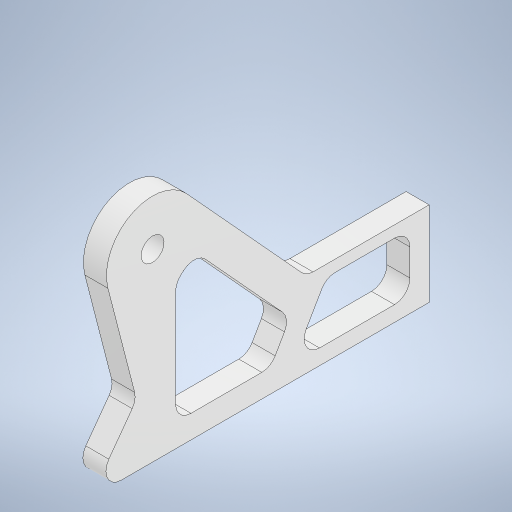
# Autodesk Inventor part: Upright
Saved by Autodesk Inventor 2023.2 (Build 272271000, 271)
## iProperties
Created: 2023-11-13
Part Number: Upright
Material: UHMW, White
Document SubType Name: Modeling
Designer: Nathan Cai
Density: 0.94 g/cm^3
Appearance: Smooth - White
Mass: 83.2223 g
Surface Area: 143.277 cm^2
Volume: 30.8231 cm^3
Author: Nathan Cai
Autodesk Inventor part; units mm, degrees
ref_plane "YZ Plane" through (0, 0, 0) normal (1, 0, 0) x (0, 1, 0)
ref_plane "XZ Plane" through (0, 0, 0) normal (0, 1, 0) x (-1, 0, 0)
ref_plane "XY Plane" through (0, 0, 0) normal (0, 0, 1) x (1, 0, 0)
sketch "Sketch1" plane through (0, 0, 0) normal (1, 0, 0) x (0, 1, 0)
  circle A0 centre (0, 0) radius 4.7625
  line L0 (0, 0) -> (-76.2, 0) construction
  circle A1 centre (0, 0) radius 19.05
  line L1 (-4.7625, 18.4451) -> (-76.2, 0)
  line L2 (-76.2, 0) -> (-76.2, -114.3)
  circle A2 centre (0, 0) radius 76.2 construction
  line L3 (-76.2, -114.3) -> (-41.275, -114.3)
  line L4 (-41.275, -114.3) -> (-41.275, -63.5)
  line L5 (-41.275, -63.5) -> (-76.2, -43.336)
  line L6 (-41.275, -63.5) -> (12.8474, -14.0658)
  line L7 (-52.8131, -56.8385) -> (-8.9789, -16.8012)
  line L8 (-66.675, -9.525) -> (-66.675, -48.8353)
  line L9 (-46.0375, -71.7489) -> (-76.2, -54.3346)
  line L10 (-46.0375, -71.7489) -> (-46.0375, -106.3625)
  line L11 (-46.0375, -106.3625) -> (-69.85, -106.3625)
  line L12 (-69.85, -106.3625) -> (-69.85, -58.0007)
  line L13 (-66.675, -9.525) -> (-64.7847, -9.525)
  line L14 (-64.7847, -9.525) -> (-16.4978, -9.525)
  line L15 (-76.2, 0) -> (-41.275, 0)
  line L16 (-41.275, 0) -> (-41.275, 25.4) construction
  line L17 (-41.275, 25.4) -> (-76.2, 25.4) construction
  line L18 (-76.2, 25.4) -> (-76.2, 0)
  line L19 (-41.275, 0) -> (-76.2, 25.4)
  point P0 (-50.4255, 6.6549)
  dimension "d0" = 9.525
  dimension "d1" = 76.2
  dimension "d2" = 38.1
  dimension "d3" = 114.3
  dimension "d4" = 152.4
  dimension "d5" = 34.925
  dimension "d6" = 50.8
  dimension "d7" = 60
  dimension "d9" = 12.7
  dimension "d10" = 9.525
  dimension "d11" = 9.525
  dimension "d12" = 7.9375
  dimension "d13" = 6.35
  dimension "d14" = 4.7625
  dimension "d17" = 9.525
  dimension "d19" = 34.925
  dimension "d20" = 25.4
  constraints: 40 end point, 6 parallel, 6 point on line, 4 point on circle, 3 centre point, 3 coincident, 3 horizontal, 3 perpendicular, 2 tangent, 1 vertical
  measures "d0" diameter of A0
  measures "d1" distance of L0.start L0.end
  measures "d2" diameter of A1
  measures "d3" distance of L0.end L2.end
  measures "d4" diameter of A2
  measures "d5" distance of L2.end L3.end
  measures "d6" distance of L3.end L4.end
  measures "d7" angle of L2 L5
  measures "d9" distance between parallel lines of L6 L7
  measures "d10" distance between parallel lines of L2 L8
  measures "d11" distance between parallel lines of L5 L9
  measures "d12" distance between parallel lines of L3 L11
  measures "d13" distance between parallel lines of L2 L12
  measures "d14" distance between parallel lines of L4 L10
  measures "d17" distance from line of L0 L8.start
  measures "d19" distance of L17.end L16.end
  measures "d20" distance of L16.end L15.end
extrude "Extrusion1" add sketch "Sketch1" along normal blind 9.525 contours A1 | A1 L14 L13 L8 L5 L2 L15 L19 L1 | L6 L5 L7 A1 | L19 L15 L1 | L1 L18 L19 | L4 L3 L2 L5
fillet "Fillet1" radius 6.35 10 edges at (4.7625, -8.9789, -16.8012) (4.7625, -16.4978, -9.525) (4.7625, -52.8131, -56.8385) (4.7625, -66.675, -9.525) (4.7625, -66.675, -48.8353) (4.7625, -69.85, -58.0007) (4.7625, -46.0375, -71.7489) (4.7625, -46.0375, -106.3625) (4.7625, -69.85, -106.3625) (4.7625, -41.275, -63.5)
fillet "Fillet2" radius 6.35 2 edges at (4.7625, -76.2, 25.4) (4.7625, -50.4255, 6.6549)
sketch "Sketch2" plane through (0, 0, 0) normal (-1, 0, 0) x (0, 0, 1)
  circle A0 centre (0, 0) radius 11.1125
  dimension "d24" = 22.225
  constraints: 1 centre point, 1 coincident
  measures "d24" diameter of A0
extrude "Extrusion2" cut sketch "Sketch2" against normal blind 1.5875
equation "\"d9\" = d8"
equation "\"d8\" = 12.7"
body "Solid1"
